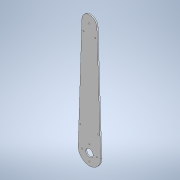
# Autodesk Inventor part: 関節2_側板1
Saved by Autodesk Inventor 2021 (Build 250183000, 183)
## iProperties
Created: 2022-02-02
Part Number: 関節2_側板1
Material: 一般
Document SubType Name: Modeling
Designer: hirohumi
Density: 1 g/cm^3
Appearance: 既定
Author: hirohumi
Autodesk Inventor part; units mm, degrees
ref_plane "YZ Plane" through (0, 0, 0) normal (1, 0, 0) x (0, 1, 0)
ref_plane "XZ Plane" through (0, 0, 0) normal (0, 1, 0) x (-1, 0, 0)
ref_plane "XY Plane" through (0, 0, 0) normal (0, 0, 1) x (1, 0, 0)
sketch "スケッチ1" plane through (0, 0, 0) normal (0, 0, 1) x (1, 0, 0)
  circle A0 centre (0, 0) radius 10
  circle A1 centre (0, 300) radius 1.6
  circle A2 centre (0, 0) radius 20 construction
  circle A3 centre (0, 20) radius 1.6
  circle A4 centre (20, 0) radius 1.6
  circle A5 centre (0, -20) radius 1.6
  circle A6 centre (-20, 0) radius 1.6
  arc A7 (19.9889, 300.6667) -> (-19.9889, 300.6667) centre (0, 300) ccw
  arc A8 (-29.9833, 1) -> (29.9833, 1) centre (0, 0) ccw
  line L0 (-19.9889, 300.6667) -> (-29.9833, 1)
  line L1 (19.9889, 300.6667) -> (29.9833, 1)
  circle A9 centre (0, 300) radius 30 construction
  circle A10 centre (0, 0) radius 60 construction
  circle A11 centre (-24.1831, 54.9106) radius 1.6
  circle A12 centre (24.1831, 54.9106) radius 1.6
  circle A13 centre (-15.8577, 274.5337) radius 1.6
  circle A14 centre (15.8577, 274.5337) radius 1.6
  circle A15 centre (0, 0) radius 13 construction
  circle A16 centre (0, 300) radius 25 construction
  line L2 (-24.98, 299) -> (-12.9896, -0.52) construction
  dimension "d20" = 26
  dimension "d21" = 50
  dimension "d0" = 20
  dimension "d1" = 3.2
  dimension "d2" = 300
  dimension "d3" = 40
  dimension "d4" = 3.2
  dimension "d5" = 3.2
  dimension "d6" = 3.2
  dimension "d7" = 3.2
  dimension "d8" = 20
  dimension "d9" = 30
  dimension "d10" = 60
  dimension "d11" = 120
  dimension "d12" = 3.2
  dimension "d13" = 3.2
  dimension "d14" = 3.2
  dimension "d15" = 3.2
  dimension "d16" = 5
  dimension "d17" = 4
  constraints: 15 centre point, 12 point on circle, 8 coincident, 6 end point, 4 horizontal alignment, 4 tangent, 3 vertical alignment, 8 other
  measures "d0" diameter of A0
  measures "d1" diameter of A1
  measures "d2" distance of point (0, 0) A1.centre
  measures "d3" diameter of A2
  measures "d4" diameter of A3
  measures "d5" diameter of A4
  measures "d6" diameter of A5
  measures "d7" diameter of A6
  measures "d8" radius of A7
  measures "d9" radius of A8
  measures "d10" diameter of A9
  measures "d11" diameter of A10
  measures "d12" diameter of A11
  measures "d13" diameter of A12
  measures "d14" diameter of A13
  measures "d15" diameter of A14
  measures "d16" distance from line of L0 A13.centre
  measures "d17" distance from line of L1 A12.centre
extrude "押し出し1" add sketch "スケッチ1" along normal blind 3
